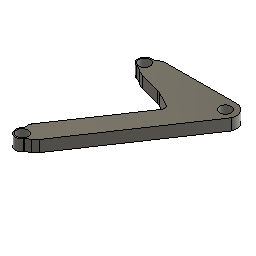
final (Autodesk Fusion 360 design; units mm, degrees)
Autodesk Fusion 360 part; units mm, degrees
other "Base Mesh Feature1"
sketch "Sketch1" plane through (0, 0, 0) normal (0, 1, 0) x (1, 0, 0)
  circle A0 centre (2, 28) radius 1
  circle A1 centre (2, 6.6) radius 1
  circle A2 centre (16.2, 28) radius 1
  line L0 (4.4281, 7.132) -> (17.9902, 27.3043)
  line L1 (10.5362, 22.356) -> (1.3727, 8.8076)
  line L2 (3.5142, 29.8509) -> (16.0424, 29.9142)
  spline S0 degree 5 poles (1.2472, 28.8931) (1.2627, 28.9154) (1.2944, 28.958) (1.3437, 29.0159) (1.4134, 29.0807) (1.5069, 29.1412) (1.6068, 29.1823) (1.713, 29.2058) (1.8253, 29.2157) (1.9428, 29.2182) (2.065, 29.2204) (2.1906, 29.2292) (2.3185, 29.2503) (2.4474, 29.2865) (2.5756, 29.3376) (2.7017, 29.4005) (2.8243, 29.471) (2.9421, 29.5444) (3.0541, 29.6165) (3.1597, 29.6845) (3.2422, 29.7364) (3.3015, 29.7726) (3.3405, 29.7959) (3.361, 29.8079) (3.3639, 29.8096) knots 0 0 0 0 0 0 0.05 0.1 0.15 0.2 0.25 0.3 0.35 0.4 0.45 0.5 0.55 0.6 0.65 0.7 0.75 0.8 0.85 0.9 0.95 0.958194 0.958194 0.958194 0.958194 0.958194 0.958194
  line L3 (10.5, 23.4) -> (7.7962, 24.7985)
  line L4 (7.3864, 24.9562) -> (3.8, 25.9)
  spline S1 degree 5 poles (1.3727, 8.8076) (1.3563, 8.7894) (1.3253, 8.7531) (1.2846, 8.6984) (1.2417, 8.625) (1.2069, 8.5324) (1.1906, 8.4392) (1.1913, 8.3454) (1.2062, 8.2512) (1.2309, 8.1568) (1.2591, 8.0627) (1.2843, 7.9695) (1.3005, 7.8782) (1.3033, 7.7899) (1.2912, 7.7062) (1.2663, 7.629) (1.2329, 7.5605) (1.1968, 7.5029) (1.1636, 7.4579) (1.1381, 7.4271) (1.1229, 7.4109) (1.12, 7.4099) (1.1231, 7.4157) (1.1275, 7.4226) (1.1303, 7.4268) knots 0 0 0 0 0 0 0.05 0.1 0.15 0.2 0.25 0.3 0.35 0.4 0.45 0.5 0.55 0.6 0.65 0.7 0.75 0.8 0.85 0.9 0.95 1 1 1 1 1 1
  spline S2 degree 5 poles (3.6859, 6.4708) (3.672, 6.4635) (3.6408, 6.4473) (3.5918, 6.421) (3.5243, 6.3827) (3.4383, 6.3282) (3.3498, 6.2651) (3.2639, 6.1967) (3.1832, 6.126) (3.1103, 6.0569) (3.0477, 5.9933) (2.9974, 5.9392) (2.9611, 5.8973) (2.9394, 5.8691) (2.9339, 5.858) (2.9364, 5.8561) (2.9411, 5.8578) (2.9441, 5.8593) knots 0.358952 0.358952 0.358952 0.358952 0.358952 0.358952 0.4 0.45 0.5 0.55 0.6 0.65 0.7 0.75 0.8 0.85 0.9 0.95 1 1 1 1 1 1
  arc A3 (3.6859, 6.4708) -> (4.4281, 7.132) centre (2.7684, 8.2478) ccw
  spline S3 degree 5 poles (10.5, 23.4) (10.5129, 23.3836) (10.5393, 23.3484) (10.5766, 23.2931) (10.62, 23.2162) (10.6618, 23.1159) (10.6904, 23.0105) (10.7038, 22.9031) (10.7015, 22.7946) (10.6836, 22.6854) (10.6504, 22.5758) (10.6119, 22.488) (10.5766, 22.422) (10.5501, 22.378) (10.5362, 22.356) knots 0.340646 0.340646 0.340646 0.340646 0.340646 0.340646 0.4 0.466667 0.533333 0.6 0.666667 0.733333 0.8 0.866667 0.933333 1 1 1 1 1 1
  line L5 (10.429, 23.4902) -> (10.571, 23.3098)
  arc A4 (1.2472, 28.8931) -> (1.8086, 26.8478) centre (2, 28) ccw
  spline S4 degree 5 poles (2.7764, 26.3984) (2.7843, 26.396) (2.7984, 26.3908) (2.8142, 26.3823) (2.8273, 26.3691) (2.8431, 26.347) (2.8736, 26.3167) (2.9333, 26.2757) (3.0301, 26.2228) (3.1657, 26.1583) (3.3393, 26.0829) (3.5067, 26.0144) (3.6475, 25.9589) (3.7481, 25.9199) (3.8, 25.9) knots 0 0 0 0 0 0 0.1 0.2 0.3 0.4 0.5 0.6 0.7 0.8 0.9 1 1 1 1 1 1
  line L6 (2.6004, 26.6214) -> (3.0473, 26.4827)
  arc A5 (17.5199, 26.6047) -> (16.0424, 29.9142) centre (16.2, 28) ccw
  arc A6 (2.7764, 26.3984) -> (1.8086, 26.8478) centre (1.4808, 24.8748) ccw
  arc A7 (7.7962, 24.7985) -> (7.3864, 24.9562) centre (6.8774, 23.0221) ccw
  arc A8 (3.5142, 29.8509) -> (3.3639, 29.8096) centre (3.5157, 29.5509) ccw
  arc A9 (1.168, 7.4648) -> (3.0105, 5.9527) centre (2, 6.6) ccw
  point P0 (1.7, 29.2)
  point P1 (2.3, 29.25)
  point P2 (2.95, 29.55)
  point P3 (10.7, 22.9)
  point P4 (2.9, 26.3)
  point P5 (1.2, 8.3)
  point P6 (1.3, 7.8)
  point P7 (3.4, 6.3)
  dimension "d1" = 2
  dimension "d2" = 2
  dimension "d3" = 2
  dimension "d4" = 2
  dimension "d5" = 2
  dimension "d6" = 2
  dimension "d7" = 0.3
  constraint concentric A0 A4
  constraint concentric A2 A5
  constraint concentric A1 A9
  constraint coincident L0.end A5
  constraint coincident L3.start S3.start
  constraint coincident S1.end A9
  constraint coincident S2.end A9
  constraint tangent L0 A3
  constraint tangent S2 A3
  constraint midpoint L3.start L5
  constraint coincident L0 A5.start
  constraint tangent A4 A6
  constraint tangent S4 A6
  constraint tangent L3 A7
  constraint tangent L4 A7
  constraint tangent L2 A8
  constraint tangent S0 A8
  measures "d1" diameter of A0
  measures "d2" diameter of A1
  measures "d3" diameter of A2
  measures "d4" radius of A3
  measures "d5" radius of A6
  measures "d6" radius of A7
  measures "d7" radius of A8
extrude "Extrude1" add sketch "Sketch1" along normal blind 2 contours L0 L1 L2 S0 L3 L4 S1 S2 A3 S3 A4 S4 A5 A6 A7 A8 A9
